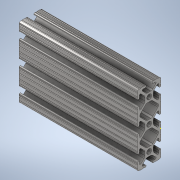
# Autodesk Inventor part: 5in 3x1 T slot
Saved by Autodesk Inventor 2020 (Build 240168000, 168)
## iProperties
Created: 2020-01-12
Part Number: 5in 3x1 T slot
Material: Steel, Alloy
Document SubType Name: Modeling
Designer: Michael
Density: 7.73 g/cm^3
Appearance: Semi-Polished
Author: Michael
Autodesk Inventor part; units mm, degrees
ref_plane "YZ Plane" through (0, 0, 0) normal (1, 0, 0) x (0, 1, 0)
ref_plane "XZ Plane" through (0, 0, 0) normal (0, 1, 0) x (-1, 0, 0)
ref_plane "XY Plane" through (0, 0, 0) normal (0, 0, 1) x (1, 0, 0)
sketch "Sketch1" plane through (0, 0, 0) normal (1, 0, 0) x (0, 1, 0)
  arc A0 (-28.0416, 5.8674) -> (-28.0416, 6.8834) centre (-28.0416, 6.3754) ccw
  line L0 (-28.0416, 7.8897) -> (-28.0416, 6.8834)
  arc A1 (-25.8318, 7.8897) -> (-28.0416, 7.8897) centre (-26.9367, 7.8897) ccw
  line L1 (-25.8318, 5.7172) -> (-25.8318, 7.8897)
  arc A2 (16.5332, 1.7018) -> (17.2516, 3.4362) centre (16.5332, 2.7178) ccw
  line L2 (16.383, -0.508) -> (19.6088, -0.508)
  arc A3 (16.383, -0.508) -> (15.367, -0.508) centre (15.875, -0.508) ccw
  line L3 (13.9343, 6.7536) -> (17.2516, 3.4362)
  line L4 (16.5332, 1.7018) -> (14.3607, 1.7018)
  line L5 (14.3607, -0.508) -> (15.367, -0.508)
  arc A4 (14.3607, 1.7018) -> (14.3607, -0.508) centre (14.3607, 0.5969) ccw
  arc A5 (20.6248, -0.508) -> (19.6088, -0.508) centre (20.1168, -0.508) ccw
  arc A6 (44.2142, 4.9988) -> (45.9486, 5.7172) centre (44.9326, 5.7172) ccw
  arc A7 (41.9332, 1.7018) -> (42.6516, 3.4362) centre (41.9332, 2.7178) ccw
  line L6 (41.783, -0.508) -> (45.0088, -0.508)
  arc A8 (41.783, -0.508) -> (40.767, -0.508) centre (41.275, -0.508) ccw
  line L7 (39.7607, -0.508) -> (40.767, -0.508)
  arc A9 (39.7607, 1.7018) -> (39.7607, -0.508) centre (39.7607, 0.5969) ccw
  line L8 (41.9332, 1.7018) -> (39.7607, 1.7018)
  line L9 (39.3343, 6.7536) -> (42.6516, 3.4362)
  line L10 (44.2142, 4.9988) -> (40.8968, 8.3161)
  arc A10 (39.3343, 6.7536) -> (37.0892, 7.6835) centre (37.0892, 4.5085) ccw
  line L11 (45.9486, 7.8897) -> (45.9486, 5.7172)
  arc A11 (45.9486, 18.6668) -> (44.2142, 19.3852) centre (44.9326, 18.6668) ccw
  line L12 (40.8968, 16.0679) -> (44.2142, 19.3852)
  line L13 (48.1584, 18.5166) -> (48.1584, 21.7424)
  line L14 (42.6516, 20.9478) -> (39.3343, 17.6304)
  arc A12 (48.1584, 22.7584) -> (48.1584, 21.7424) centre (48.1584, 22.2504) ccw
  arc A13 (48.1584, 22.7584) -> (46.0248, 24.892) centre (46.0504, 22.784) ccw
  line L15 (39.7607, 22.6822) -> (41.9332, 22.6822)
  line L16 (45.0088, 24.892) -> (41.783, 24.892)
  arc A14 (45.0088, 24.892) -> (46.0248, 24.892) centre (45.5168, 24.892) ccw
  line L17 (40.767, 24.892) -> (39.7607, 24.892)
  arc A15 (39.7607, 24.892) -> (39.7607, 22.6822) centre (39.7607, 23.7871) ccw
  arc A16 (40.767, 24.892) -> (41.783, 24.892) centre (41.275, 24.892) ccw
  line L18 (24.892, 24.892) -> (20.6248, 24.892)
  arc A17 (24.892, 24.892) -> (25.908, 24.892) centre (25.4, 24.892) ccw
  line L19 (29.1338, 24.892) -> (25.908, 24.892)
  arc A18 (28.9836, 22.6822) -> (28.2652, 20.9478) centre (28.9836, 21.6662) ccw
  arc A19 (29.1338, 24.892) -> (30.1498, 24.892) centre (29.6418, 24.892) ccw
  line L20 (28.9836, 22.6822) -> (31.1561, 22.6822)
  line L21 (31.1561, 24.892) -> (30.1498, 24.892)
  arc A20 (31.1561, 22.6822) -> (31.1561, 24.892) centre (31.1561, 23.7871) ccw
  arc A21 (-0.508, 24.892) -> (0.508, 24.892) centre (0, 24.892) ccw
  line L22 (3.7338, 24.892) -> (0.508, 24.892)
  arc A22 (3.5836, 22.6822) -> (2.8652, 20.9478) centre (3.5836, 21.6662) ccw
  arc A23 (3.7338, 24.892) -> (4.7498, 24.892) centre (4.2418, 24.892) ccw
  line L23 (3.5836, 22.6822) -> (5.7561, 22.6822)
  line L24 (5.7561, 24.892) -> (4.7498, 24.892)
  arc A24 (5.7561, 22.6822) -> (5.7561, 24.892) centre (5.7561, 23.7871) ccw
  arc A25 (-0.9743, 21.6622) -> (-2.0879, 22.1234) centre (-2.0879, 20.5486) ccw
  arc A26 (5.5499, 13.8228) -> (4.62, 16.0679) centre (2.3749, 13.8228) ccw
  line L25 (-2.0879, 22.1234) -> (-3.1953, 22.1234)
  arc A27 (-3.1953, 22.1234) -> (-4.3089, 21.6622) centre (-3.1953, 20.5486) ccw
  line L26 (5.5499, 10.5612) -> (5.5499, 13.8228)
  arc A28 (4.62, 8.3161) -> (5.5499, 10.5612) centre (2.3749, 10.5612) ccw
  line L27 (-4.3089, 21.6622) -> (-9.9032, 16.0679)
  line L28 (-8.1484, 20.9478) -> (-11.4657, 17.6304)
  arc A29 (-9.9032, 16.0679) -> (-10.8331, 13.8228) centre (-7.6581, 13.8228) ccw
  line L29 (-10.8331, 13.8228) -> (-10.8331, 10.5612)
  arc A30 (-10.8331, 10.5612) -> (-9.9032, 8.3161) centre (-7.6581, 10.5612) ccw
  line L30 (-21.6662, 24.892) -> (-24.892, 24.892)
  arc A31 (-21.8164, 22.6822) -> (-22.5348, 20.9478) centre (-21.8164, 21.6662) ccw
  arc A32 (-21.6662, 24.892) -> (-20.6502, 24.892) centre (-21.1582, 24.892) ccw
  line L31 (-19.6439, 24.892) -> (-20.6502, 24.892)
  arc A33 (-19.6439, 22.6822) -> (-19.6439, 24.892) centre (-19.6439, 23.7871) ccw
  line L32 (-24.0974, 19.3852) -> (-20.78, 16.0679)
  line L33 (-19.2175, 17.6304) -> (-22.5348, 20.9478)
  arc A34 (-19.2175, 17.6304) -> (-16.9724, 16.7005) centre (-16.9724, 19.8755) ccw
  line L34 (-21.8164, 22.6822) -> (-19.6439, 22.6822)
  line L35 (-3.1953, 2.2606) -> (-2.0879, 2.2606)
  line L36 (-4.7752, -0.508) -> (-0.508, -0.508)
  arc A35 (-4.3089, 2.7218) -> (-3.1953, 2.2606) centre (-3.1953, 3.8354) ccw
  arc A36 (-4.7752, -0.508) -> (-5.7912, -0.508) centre (-5.2832, -0.508) ccw
  arc A37 (-8.8668, 1.7018) -> (-8.1484, 3.4362) centre (-8.8668, 2.7178) ccw
  line L37 (-9.9032, 8.3161) -> (-4.3089, 2.7218)
  line L38 (-11.4657, 6.7536) -> (-8.1484, 3.4362)
  arc A38 (-9.017, -0.508) -> (-10.033, -0.508) centre (-9.525, -0.508) ccw
  line L39 (-8.8668, 1.7018) -> (-11.0393, 1.7018)
  line L40 (-11.0393, -0.508) -> (-10.033, -0.508)
  arc A39 (-11.0393, 1.7018) -> (-11.0393, -0.508) centre (-11.0393, 0.5969) ccw
  line L41 (-9.017, -0.508) -> (-5.7912, -0.508)
  arc A40 (-20.78, 8.3161) -> (-19.8501, 10.5612) centre (-23.0251, 10.5612) ccw
  arc A41 (-28.0416, 16.4943) -> (-25.8318, 16.4943) centre (-26.9367, 16.4943) ccw
  arc A42 (-16.9724, 7.6835) -> (-19.2175, 6.7536) centre (-16.9724, 4.5085) ccw
  line L42 (-19.8501, 13.8228) -> (-19.8501, 10.5612)
  arc A43 (-19.8501, 13.8228) -> (-20.78, 16.0679) centre (-23.0251, 13.8228) ccw
  line L43 (-16.9724, 7.6835) -> (-13.7108, 7.6835)
  arc A44 (-11.4657, 6.7536) -> (-13.7108, 7.6835) centre (-13.7108, 4.5085) ccw
  circle A45 centre (-15.3416, 12.192) radius 2.6035
  arc A46 (-13.7108, 16.7005) -> (-11.4657, 17.6304) centre (-13.7108, 19.8755) ccw
  line L44 (-13.7108, 16.7005) -> (-16.9724, 16.7005)
  line L45 (6.1825, 17.6304) -> (2.8652, 20.9478)
  line L46 (4.62, 16.0679) -> (-0.9743, 21.6622)
  line L47 (20.6248, -0.508) -> (24.892, -0.508)
  arc A47 (25.908, -0.508) -> (24.892, -0.508) centre (25.4, -0.508) ccw
  arc A48 (28.2652, 3.4362) -> (28.9836, 1.7018) centre (28.9836, 2.7178) ccw
  line L48 (25.908, -0.508) -> (29.1338, -0.508)
  arc A49 (30.1498, -0.508) -> (29.1338, -0.508) centre (29.6418, -0.508) ccw
  line L49 (31.1561, 1.7018) -> (28.9836, 1.7018)
  line L50 (30.1498, -0.508) -> (31.1561, -0.508)
  arc A50 (31.1561, -0.508) -> (31.1561, 1.7018) centre (31.1561, 0.5969) ccw
  line L51 (28.2652, 3.4362) -> (31.5825, 6.7536)
  arc A51 (48.1584, 7.8897) -> (45.9486, 7.8897) centre (47.0535, 7.8897) ccw
  line L52 (48.1584, 6.8834) -> (48.1584, 7.8897)
  arc A52 (48.1584, 6.8834) -> (48.1584, 5.8674) centre (48.1584, 6.3754) ccw
  line L53 (48.1584, 2.6416) -> (48.1584, 5.8674)
  arc A53 (46.0248, -0.508) -> (45.0088, -0.508) centre (45.5168, -0.508) ccw
  arc A54 (48.1584, 2.6416) -> (48.1584, 1.6256) centre (48.1584, 2.1336) ccw
  arc A55 (46.0248, -0.508) -> (48.1584, 1.6256) centre (46.0504, 1.6) ccw
  line L54 (45.9486, 18.6668) -> (45.9486, 16.4943)
  arc A56 (48.1584, 18.5166) -> (48.1584, 17.5006) centre (48.1584, 18.0086) ccw
  line L55 (48.1584, 16.4943) -> (48.1584, 17.5006)
  arc A57 (45.9486, 16.4943) -> (48.1584, 16.4943) centre (47.0535, 16.4943) ccw
  arc A58 (33.8276, 7.6835) -> (31.5825, 6.7536) centre (33.8276, 4.5085) ccw
  line L56 (33.8276, 7.6835) -> (37.0892, 7.6835)
  arc A59 (39.9669, 10.5612) -> (40.8968, 8.3161) centre (43.1419, 10.5612) ccw
  line L57 (39.9669, 10.5612) -> (39.9669, 13.8228)
  arc A60 (40.8968, 16.0679) -> (39.9669, 13.8228) centre (43.1419, 13.8228) ccw
  circle A61 centre (35.4584, 12.192) radius 2.6035
  line L58 (30.9499, 10.5612) -> (30.9499, 13.8228)
  arc A62 (37.0892, 16.7005) -> (39.3343, 17.6304) centre (37.0892, 19.8755) ccw
  arc A63 (42.6516, 20.9478) -> (41.9332, 22.6822) centre (41.9332, 21.6662) ccw
  line L59 (37.0892, 16.7005) -> (33.8276, 16.7005)
  arc A64 (31.5825, 17.6304) -> (33.8276, 16.7005) centre (33.8276, 19.8755) ccw
  line L60 (31.5825, 17.6304) -> (28.2652, 20.9478)
  arc A65 (19.6088, 24.892) -> (20.6248, 24.892) centre (20.1168, 24.892) ccw
  arc A66 (17.2516, 20.9478) -> (16.5332, 22.6822) centre (16.5332, 21.6662) ccw
  line L61 (19.6088, 24.892) -> (16.383, 24.892)
  arc A67 (15.367, 24.892) -> (16.383, 24.892) centre (15.875, 24.892) ccw
  line L62 (15.367, 24.892) -> (14.3607, 24.892)
  line L63 (14.3607, 22.6822) -> (16.5332, 22.6822)
  arc A68 (14.3607, 24.892) -> (14.3607, 22.6822) centre (14.3607, 23.7871) ccw
  arc A69 (8.4276, 7.6835) -> (6.1825, 6.7536) centre (8.4276, 4.5085) ccw
  line L64 (8.4276, 7.6835) -> (11.6892, 7.6835)
  arc A70 (13.9343, 6.7536) -> (11.6892, 7.6835) centre (11.6892, 4.5085) ccw
  arc A71 (6.1825, 17.6304) -> (8.4276, 16.7005) centre (8.4276, 19.8755) ccw
  circle A72 centre (10.0584, 12.192) radius 2.6035
  line L65 (11.6892, 16.7005) -> (8.4276, 16.7005)
  arc A73 (11.6892, 16.7005) -> (13.9343, 17.6304) centre (11.6892, 19.8755) ccw
  line L66 (-0.508, 24.892) -> (-4.7752, 24.892)
  arc A74 (-5.7912, 24.892) -> (-4.7752, 24.892) centre (-5.2832, 24.892) ccw
  line L67 (-5.7912, 24.892) -> (-9.017, 24.892)
  arc A75 (-8.1484, 20.9478) -> (-8.8668, 22.6822) centre (-8.8668, 21.6662) ccw
  arc A76 (-10.033, 24.892) -> (-9.017, 24.892) centre (-9.525, 24.892) ccw
  line L68 (-11.0393, 22.6822) -> (-8.8668, 22.6822)
  line L69 (-10.033, 24.892) -> (-11.0393, 24.892)
  arc A77 (-11.0393, 24.892) -> (-11.0393, 22.6822) centre (-11.0393, 23.7871) ccw
  arc A78 (-24.0974, 19.3852) -> (-25.8318, 18.6668) centre (-24.8158, 18.6668) ccw
  line L70 (-25.8318, 16.4943) -> (-25.8318, 18.6668)
  line L71 (-28.0416, 17.5006) -> (-28.0416, 16.4943)
  arc A79 (-28.0416, 17.5006) -> (-28.0416, 18.5166) centre (-28.0416, 18.0086) ccw
  line L72 (-28.0416, 21.7424) -> (-28.0416, 18.5166)
  arc A80 (-25.908, 24.892) -> (-24.892, 24.892) centre (-25.4, 24.892) ccw
  arc A81 (-28.0416, 21.7424) -> (-28.0416, 22.7584) centre (-28.0416, 22.2504) ccw
  arc A82 (-25.908, 24.892) -> (-28.0416, 22.7584) centre (-25.9336, 22.784) ccw
  arc A83 (-25.8318, 5.7172) -> (-24.0974, 4.9988) centre (-24.8158, 5.7172) ccw
  line L73 (-20.78, 8.3161) -> (-24.0974, 4.9988)
  line L74 (-28.0416, 5.8674) -> (-28.0416, 2.6416)
  arc A84 (-28.0416, 1.6256) -> (-28.0416, 2.6416) centre (-28.0416, 2.1336) ccw
  arc A85 (-28.0416, 1.6256) -> (-25.908, -0.508) centre (-25.9336, 1.6) ccw
  line L75 (-22.5348, 3.4362) -> (-19.2175, 6.7536)
  arc A86 (-22.5348, 3.4362) -> (-21.8164, 1.7018) centre (-21.8164, 2.7178) ccw
  arc A87 (-24.892, -0.508) -> (-25.908, -0.508) centre (-25.4, -0.508) ccw
  line L76 (-24.892, -0.508) -> (-21.6662, -0.508)
  line L77 (-19.6439, 1.7018) -> (-21.8164, 1.7018)
  arc A88 (-20.6502, -0.508) -> (-21.6662, -0.508) centre (-21.1582, -0.508) ccw
  line L78 (-20.6502, -0.508) -> (-19.6439, -0.508)
  arc A89 (-19.6439, -0.508) -> (-19.6439, 1.7018) centre (-19.6439, 0.5969) ccw
  arc A90 (23.3121, 2.2606) -> (24.4257, 2.7218) centre (23.3121, 3.8354) ccw
  arc A91 (30.02, 8.3161) -> (30.9499, 10.5612) centre (27.7749, 10.5612) ccw
  line L79 (24.4257, 2.7218) -> (30.02, 8.3161)
  line L80 (22.2047, 2.2606) -> (23.3121, 2.2606)
  arc A92 (21.0911, 2.7218) -> (22.2047, 2.2606) centre (22.2047, 3.8354) ccw
  arc A93 (30.9499, 13.8228) -> (30.02, 16.0679) centre (27.7749, 13.8228) ccw
  line L81 (15.4968, 8.3161) -> (21.0911, 2.7218)
  line L82 (30.02, 16.0679) -> (24.4257, 21.6622)
  arc A94 (14.5669, 10.5612) -> (15.4968, 8.3161) centre (17.7419, 10.5612) ccw
  line L83 (14.5669, 13.8228) -> (14.5669, 10.5612)
  arc A95 (24.4257, 21.6622) -> (23.3121, 22.1234) centre (23.3121, 20.5486) ccw
  line L84 (23.3121, 22.1234) -> (22.2047, 22.1234)
  arc A96 (22.2047, 22.1234) -> (21.0911, 21.6622) centre (22.2047, 20.5486) ccw
  arc A97 (15.4968, 16.0679) -> (14.5669, 13.8228) centre (17.7419, 13.8228) ccw
  line L85 (21.0911, 21.6622) -> (15.4968, 16.0679)
  line L86 (17.2516, 20.9478) -> (13.9343, 17.6304)
  arc A98 (-2.0879, 2.2606) -> (-0.9743, 2.7218) centre (-2.0879, 3.8354) ccw
  arc A99 (0.508, -0.508) -> (-0.508, -0.508) centre (0, -0.508) ccw
  line L87 (-0.9743, 2.7218) -> (4.62, 8.3161)
  line L88 (0.508, -0.508) -> (3.7338, -0.508)
  arc A100 (2.8652, 3.4362) -> (3.5836, 1.7018) centre (3.5836, 2.7178) ccw
  arc A101 (4.7498, -0.508) -> (3.7338, -0.508) centre (4.2418, -0.508) ccw
  line L89 (4.7498, -0.508) -> (5.7561, -0.508)
  line L90 (5.7561, 1.7018) -> (3.5836, 1.7018)
  arc A102 (5.7561, -0.508) -> (5.7561, 1.7018) centre (5.7561, 0.5969) ccw
  line L91 (2.8652, 3.4362) -> (6.1825, 6.7536)
  point P0 (0, 0)
  point P1 (-0.508, -0.508)
  point P2 (10.0584, 12.192)
  constraints: 200 point on circle, 184 end point, 103 centre point
extrude "Extrusion1" add sketch "Sketch1" along normal blind 127
sketch "Sketch2" plane through (127, 0, 0) normal (1, 0, 0) x (0, 0, -1)
  point P0 (0, 0)
body "Solid1"
